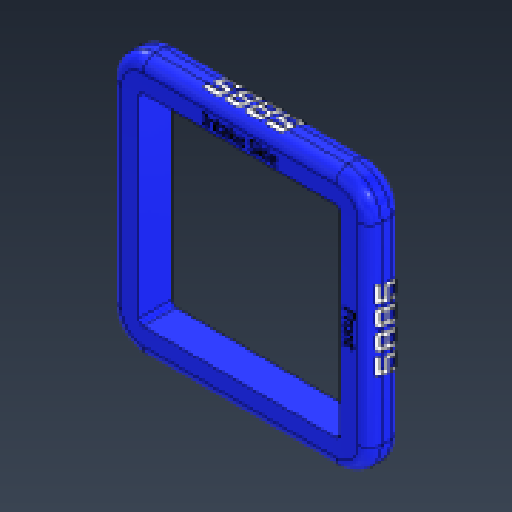
# Autodesk Inventor part: Bumpers
Saved by Autodesk Inventor 2026 (Build 300175050, 175E)
## iProperties
Created: 2026-01-21
Part Number: Bumpers
Material: Spruce
Document SubType Name: Modeling
Designer: Jthib
Mass: 13460.1 g
Surface Area: 12229.9 cm^2
Volume: 33650.4 cm^3
Density: 0.4 g/cm^3
Appearance: Blue - Wall Paint - Glossy
Author: Jthib
Autodesk Inventor part; units mm, degrees
ref_plane "YZ Plane" through (0, 0, 0) normal (1, 0, 0) x (0, 1, 0)
ref_plane "XZ Plane" through (0, 0, 0) normal (0, 1, 0) x (-1, 0, 0)
ref_plane "XY Plane" through (0, 0, 0) normal (0, 0, 1) x (1, 0, 0)
sketch "Sketch1" plane through (0, 0, 0) normal (0, 0, 1) x (1, 0, 0)
  line L0 (-349.25, 0) -> (-349.25, 336.55)
  line L1 (-336.55, 349.25) -> (336.55, 349.25)
  line L2 (349.25, 336.55) -> (349.25, -336.55)
  line L3 (336.55, -349.25) -> (-336.55, -349.25)
  line L4 (-349.25, -336.55) -> (-349.25, 0)
  arc A0 (-336.55, 349.25) -> (-349.25, 336.55) centre (-336.55, 336.55) ccw
  arc A1 (349.25, 336.55) -> (336.55, 349.25) centre (336.55, 336.55) ccw
  arc A2 (336.55, -349.25) -> (349.25, -336.55) centre (336.55, -336.55) ccw
  arc A3 (-349.25, -336.55) -> (-336.55, -349.25) centre (-336.55, -336.55) ccw
  point P0 (0, 0)
  point P1 (-349.25, 349.25)
  point P2 (349.25, 349.25)
  point P3 (349.25, -349.25)
  point P4 (-349.25, -349.25)
  dimension "d0" = 698.5
  dimension "d1" = 698.5
  dimension "d2" = 349.25
  dimension "d3" = 349.25
  dimension "d9" = 12.7
  constraints: 10 end point, 9 point on line, 8 point on circle, 8 tangent, 4 centre point, 4 perpendicular, 3 equal radius, 1 collinear, 1 vertical
  measures "d0" distance of point (349.25, 349.25) point (349.25, -349.25)
  measures "d1" distance of point (-349.25, 349.25) point (349.25, 349.25)
  measures "d2" distance from line of point (0, 0) L1
  measures "d3" distance from line of L2 point (0, 0)
  measures "d9" radius of A0
sketch "Sketch2" plane through (0, 0, 0) normal (0, 1, 0) x (-1, 0, 0)
  line L0 (412.75, 61.9125) -> (352.425, 61.9125)
  line L1 (352.425, 61.9125) -> (352.425, -52.3875)
  line L2 (352.425, -52.3875) -> (412.75, -52.3875)
  line L3 (454.025, -11.1125) -> (454.025, 20.6375)
  arc A0 (454.025, 20.6375) -> (412.75, 61.9125) centre (412.75, 20.6375) ccw
  arc A1 (412.75, -52.3875) -> (454.025, -11.1125) centre (412.75, -11.1125) ccw
  line L4 (0, -145.5372) -> (0, 106.4605) construction
  line L5 (352.425, 61.9125) -> (0, 61.9125) construction
  line L6 (352.425, -52.3875) -> (0, -52.3875) construction
  line L7 (-599.1936, -109.5375) -> (599.1891, -109.5375) construction
  point P0 (0, 0)
  point P1 (454.025, 61.9125)
  point P2 (349.25, 0)
  point P3 (349.25, 0)
  point P4 (352.425, 4.7625)
  dimension "d4" = 114.3
  dimension "d5" = 101.6
  dimension "d6" = 41.275
  dimension "d20" = 352.425
  dimension "d21" = 57.15
  constraints: 14 end point, 4 point on circle, 4 point on line, 4 tangent, 3 perpendicular, 2 centre point, 2 horizontal, 2 parallel, 1 equal radius, 1 midpoint, 2 other
  measures "d4" distance of L0.end L1.end
  measures "d5" distance of point (454.025, 61.913) L0.end
  measures "d6" radius of A0
  measures "d20" distance from line of point (0, 0) L1
  measures "d21" distance between parallel lines of L7 L2
sweep "Sweep1" add profiles "Sketch2" path "Sketch1" path curves L0 A0 L1 A1 L2 A2 L3 A3 L4
sketch "Sketch3" plane through (454.025, -336.55, 20.6375) normal (1, 0, 0) x (0, 0, -1)
  line L0 (-23.8125, 82.55) -> (-23.8125, 590.55) construction
  line L1 (-23.8125, 590.55) -> (65.0875, 590.55) construction
  line L2 (65.0875, 590.55) -> (65.0875, 82.55) construction
  line L3 (65.0875, 82.55) -> (-23.8125, 82.55) construction
  line L4 (-23.8125, 82.55) -> (65.0875, 590.55) construction
  spline S0 degree 2 poles (58.7375, 210.0554) (58.7375, 204.3206) (54.7166, 199.3768) (50.432, 199.3768) knots 0 0 0 1 2 2 2
  spline S1 degree 2 poles (50.432, 199.3768) (48.5863, 199.3768) (45.8178, 199.9701) knots 0 0 0 1 1 1
  line L5 (45.8178, 199.9701) -> (33.9527, 202.409)
  line L6 (33.9527, 202.409) -> (33.9527, 218.1632)
  line L7 (33.9527, 218.1632) -> (40.874, 216.713)
  spline S2 degree 2 poles (40.874, 216.713) (41.4013, 216.5811) (42.3242, 216.4493) (42.7856, 216.4493) knots 0 0 0 1 2 2 2
  spline S3 degree 2 poles (42.7856, 216.4493) (43.9062, 216.4493) (44.6972, 217.7017) (44.6972, 219.4156) knots 0 0 0 1 2 2 2
  line L8 (44.6972, 219.4156) -> (44.6972, 240.7727)
  spline S4 degree 2 poles (44.6972, 240.7727) (44.6972, 243.3434) (43.1152, 245.0573) (40.874, 245.6505) knots 0 0 0 1 2 2 2
  line L9 (40.874, 245.6505) -> (28.152, 248.3531)
  spline S5 degree 2 poles (28.152, 248.3531) (27.5588, 248.419) (26.7678, 248.5509) (26.4382, 248.5509) knots 0 0 0 1 2 2 2
  spline S6 degree 2 poles (26.4382, 248.5509) (24.3948, 248.5509) (24.3948, 245.6505) knots 0 0 0 1 1 1
  line L10 (24.3948, 245.6505) -> (24.3948, 204.4524)
  line L11 (24.3948, 204.4524) -> (-17.4625, 213.3512)
  line L12 (-17.4625, 213.3512) -> (-17.4625, 271.9514)
  line L13 (-17.4625, 271.9514) -> (-2.8949, 268.9192)
  line L14 (-2.8949, 268.9192) -> (-2.8949, 226.4028)
  line L15 (-2.8949, 226.4028) -> (11.8046, 223.2388)
  line L16 (11.8046, 223.2388) -> (11.8046, 257.186)
  spline S7 degree 2 poles (11.8046, 257.186) (11.8046, 261.8002) (15.7596, 266.0189) (19.3851, 266.0189) knots 0 0 0 1 2 2 2
  spline S8 degree 2 poles (19.3851, 266.0189) (20.9012, 266.0189) (22.615, 265.6234) knots 0 0 0 1 1 1
  line L17 (22.615, 265.6234) -> (45.4882, 260.8114)
  spline S9 degree 2 poles (45.4882, 260.8114) (52.2117, 259.3612) (58.7375, 252.374) (58.7375, 245.0573) knots 0 0 0 1 2 2 2
  line L18 (58.7375, 245.0573) -> (58.7375, 210.0554)
  spline S10 degree 2 poles (58.7375, 282.7618) (58.7375, 277.027) (54.7166, 271.9514) (50.432, 271.9514) knots 0 0 0 1 2 2 2
  spline S11 degree 2 poles (50.432, 271.9514) (48.5863, 271.9514) (45.8178, 272.5446) knots 0 0 0 1 1 1
  line L19 (45.8178, 272.5446) -> (27.6906, 276.3678)
  spline S12 degree 2 poles (27.6906, 276.3678) (23.406, 277.2907) (19.7147, 283.2232) (19.3851, 287.1782) knots 0 0 0 1 2 2 2
  spline S13 degree 2 poles (19.3851, 287.1782) (18.9896, 283.8824) (15.9574, 280.3228) (12.7275, 280.3228) knots 0 0 0 1 2 2 2
  spline S14 degree 2 poles (12.7275, 280.3228) (11.475, 280.3228) (9.7612, 280.6524) knots 0 0 0 1 1 1
  line L20 (9.7612, 280.6524) -> (-4.4769, 283.6846)
  spline S15 degree 2 poles (-4.4769, 283.6846) (-11.0026, 285.0689) (-17.4625, 292.5834) (-17.4625, 299.7683) knots 0 0 0 1 2 2 2
  line L21 (-17.4625, 299.7683) -> (-17.4625, 332.9905)
  spline S16 degree 2 poles (-17.4625, 332.9905) (-17.4625, 338.923) (-13.1779, 344.1304) (-8.8933, 344.1304) knots 0 0 0 1 2 2 2
  spline S17 degree 2 poles (-8.8933, 344.1304) (-6.6521, 344.1304) (-4.4769, 343.669) knots 0 0 0 1 1 1
  line L22 (-4.4769, 343.669) -> (9.7612, 340.6369)
  spline S18 degree 2 poles (9.7612, 340.6369) (14.5072, 339.5822) (18.9237, 334.1111) (19.3851, 330.0242) knots 0 0 0 1 2 2 2
  spline S19 degree 2 poles (19.3851, 330.0242) (19.7147, 333.3201) (22.4173, 337.4728) (25.4494, 337.4728) knots 0 0 0 1 2 2 2
  spline S20 degree 2 poles (25.4494, 337.4728) (25.9768, 337.4728) (27.0974, 337.341) (27.6906, 337.2751) knots 0 0 0 1 2 2 2
  line L23 (27.6906, 337.2751) -> (45.8178, 333.4519)
  spline S21 degree 2 poles (45.8178, 333.4519) (52.3436, 332.0676) (58.7375, 325.0804) (58.7375, 317.7637) knots 0 0 0 1 2 2 2
  line L24 (58.7375, 317.7637) -> (58.7375, 282.7618)
  spline S22 degree 2 poles (28.6135, 321.3891) (28.152, 321.5209) (27.361, 321.5209) knots 0 0 0 1 1 1
  spline S23 degree 2 poles (27.361, 321.5209) (26.1086, 321.5209) (25.1858, 320.0048) (25.1858, 318.0933) knots 0 0 0 1 2 2 2
  line L25 (25.1858, 318.0933) -> (25.1858, 296.6043)
  spline S24 degree 2 poles (25.1858, 296.6043) (25.1858, 294.3631) (26.6359, 292.122) (28.6135, 291.7924) knots 0 0 0 1 2 2 2
  line L26 (28.6135, 291.7924) -> (40.6103, 289.2875)
  spline S25 degree 2 poles (40.6103, 289.2875) (41.2036, 289.2216) (41.9946, 289.0898) (42.3242, 289.0898) knots 0 0 0 1 2 2 2
  spline S26 degree 2 poles (42.3242, 289.0898) (44.6972, 289.0898) (44.6972, 292.4516) knots 0 0 0 1 1 1
  line L27 (44.6972, 292.4516) -> (44.6972, 313.9405)
  spline S27 degree 2 poles (44.6972, 313.9405) (44.6972, 316.1817) (42.8515, 318.4228) (40.6103, 318.8843) knots 0 0 0 1 2 2 2
  line L28 (40.6103, 318.8843) -> (28.6135, 321.3891)
  spline S28 degree 2 poles (0.1373, 327.2557) (-0.4559, 327.3216) (-1.1151, 327.4535) (-1.4447, 327.4535) knots 0 0 0 1 2 2 2
  spline S29 degree 2 poles (-1.4447, 327.4535) (-3.6859, 327.4535) (-3.6859, 324.0917) knots 0 0 0 1 1 1
  line L29 (-3.6859, 324.0917) -> (-3.6859, 302.8005)
  spline S30 degree 2 poles (-3.6859, 302.8005) (-3.6859, 300.5593) (-2.1038, 298.5159) (0.1373, 298.1204) knots 0 0 0 1 2 2 2
  line L30 (0.1373, 298.1204) -> (10.9477, 295.8133)
  spline S31 degree 2 poles (10.9477, 295.8133) (11.3432, 295.7474) (12.0683, 295.6156) (12.3979, 295.6156) knots 0 0 0 1 2 2 2
  spline S32 degree 2 poles (12.3979, 295.6156) (14.3754, 295.6156) (14.3754, 298.8455) knots 0 0 0 1 1 1
  line L31 (14.3754, 298.8455) -> (14.3754, 320.4003)
  spline S33 degree 2 poles (14.3754, 320.4003) (14.3754, 322.6415) (12.8593, 324.5531) (10.9477, 324.9486) knots 0 0 0 1 2 2 2
  line L32 (10.9477, 324.9486) -> (0.1373, 327.2557)
  spline S34 degree 2 poles (58.7375, 355.2045) (58.7375, 349.4697) (54.7166, 344.3941) (50.432, 344.3941) knots 0 0 0 1 2 2 2
  spline S35 degree 2 poles (50.432, 344.3941) (48.5863, 344.3941) (45.8178, 344.9874) knots 0 0 0 1 1 1
  line L33 (45.8178, 344.9874) -> (27.6906, 348.8106)
  spline S36 degree 2 poles (27.6906, 348.8106) (23.406, 349.7334) (19.7147, 355.6659) (19.3851, 359.6209) knots 0 0 0 1 2 2 2
  spline S37 degree 2 poles (19.3851, 359.6209) (18.9896, 356.3251) (15.9574, 352.7656) (12.7275, 352.7656) knots 0 0 0 1 2 2 2
  spline S38 degree 2 poles (12.7275, 352.7656) (11.475, 352.7656) (9.7612, 353.0952) knots 0 0 0 1 1 1
  line L34 (9.7612, 353.0952) -> (-4.4769, 356.1273)
  spline S39 degree 2 poles (-4.4769, 356.1273) (-11.0026, 357.5116) (-17.4625, 365.0261) (-17.4625, 372.2111) knots 0 0 0 1 2 2 2
  line L35 (-17.4625, 372.2111) -> (-17.4625, 405.4332)
  spline S40 degree 2 poles (-17.4625, 405.4332) (-17.4625, 411.3657) (-13.1779, 416.5732) (-8.8933, 416.5732) knots 0 0 0 1 2 2 2
  spline S41 degree 2 poles (-8.8933, 416.5732) (-6.6521, 416.5732) (-4.4769, 416.1118) knots 0 0 0 1 1 1
  line L36 (-4.4769, 416.1118) -> (9.7612, 413.0796)
  spline S42 degree 2 poles (9.7612, 413.0796) (14.5072, 412.0249) (18.9237, 406.5538) (19.3851, 402.467) knots 0 0 0 1 2 2 2
  spline S43 degree 2 poles (19.3851, 402.467) (19.7147, 405.7628) (22.4173, 409.9156) (25.4494, 409.9156) knots 0 0 0 1 2 2 2
  spline S44 degree 2 poles (25.4494, 409.9156) (25.9768, 409.9156) (27.0974, 409.7837) (27.6906, 409.7178) knots 0 0 0 1 2 2 2
  line L37 (27.6906, 409.7178) -> (45.8178, 405.8946)
  spline S45 degree 2 poles (45.8178, 405.8946) (52.3436, 404.5104) (58.7375, 397.5232) (58.7375, 390.2064) knots 0 0 0 1 2 2 2
  line L38 (58.7375, 390.2064) -> (58.7375, 355.2045)
  spline S46 degree 2 poles (28.6135, 393.8318) (28.152, 393.9637) (27.361, 393.9637) knots 0 0 0 1 1 1
  spline S47 degree 2 poles (27.361, 393.9637) (26.1086, 393.9637) (25.1858, 392.4476) (25.1858, 390.536) knots 0 0 0 1 2 2 2
  line L39 (25.1858, 390.536) -> (25.1858, 369.0471)
  spline S48 degree 2 poles (25.1858, 369.0471) (25.1858, 366.8059) (26.6359, 364.5647) (28.6135, 364.2351) knots 0 0 0 1 2 2 2
  line L40 (28.6135, 364.2351) -> (40.6103, 361.7303)
  spline S49 degree 2 poles (40.6103, 361.7303) (41.2036, 361.6644) (41.9946, 361.5325) (42.3242, 361.5325) knots 0 0 0 1 2 2 2
  spline S50 degree 2 poles (42.3242, 361.5325) (44.6972, 361.5325) (44.6972, 364.8943) knots 0 0 0 1 1 1
  line L41 (44.6972, 364.8943) -> (44.6972, 386.3832)
  spline S51 degree 2 poles (44.6972, 386.3832) (44.6972, 388.6244) (42.8515, 390.8656) (40.6103, 391.327) knots 0 0 0 1 2 2 2
  line L42 (40.6103, 391.327) -> (28.6135, 393.8318)
  spline S52 degree 2 poles (0.1373, 399.6984) (-0.4559, 399.7644) (-1.1151, 399.8962) (-1.4447, 399.8962) knots 0 0 0 1 2 2 2
  spline S53 degree 2 poles (-1.4447, 399.8962) (-3.6859, 399.8962) (-3.6859, 396.5344) knots 0 0 0 1 1 1
  line L43 (-3.6859, 396.5344) -> (-3.6859, 375.2433)
  spline S54 degree 2 poles (-3.6859, 375.2433) (-3.6859, 373.0021) (-2.1038, 370.9586) (0.1373, 370.5631) knots 0 0 0 1 2 2 2
  line L44 (0.1373, 370.5631) -> (10.9477, 368.2561)
  spline S55 degree 2 poles (10.9477, 368.2561) (11.3432, 368.1901) (12.0683, 368.0583) (12.3979, 368.0583) knots 0 0 0 1 2 2 2
  spline S56 degree 2 poles (12.3979, 368.0583) (14.3754, 368.0583) (14.3754, 371.2882) knots 0 0 0 1 1 1
  line L45 (14.3754, 371.2882) -> (14.3754, 392.8431)
  spline S57 degree 2 poles (14.3754, 392.8431) (14.3754, 395.0843) (12.8593, 396.9958) (10.9477, 397.3913) knots 0 0 0 1 2 2 2
  line L46 (10.9477, 397.3913) -> (0.1373, 399.6984)
  spline S58 degree 2 poles (58.7375, 428.1086) (58.7375, 422.3739) (54.7166, 417.4301) (50.432, 417.4301) knots 0 0 0 1 2 2 2
  spline S59 degree 2 poles (50.432, 417.4301) (48.5863, 417.4301) (45.8178, 418.0234) knots 0 0 0 1 1 1
  line L47 (45.8178, 418.0234) -> (33.9527, 420.4623)
  line L48 (33.9527, 420.4623) -> (33.9527, 436.2164)
  line L49 (33.9527, 436.2164) -> (40.874, 434.7663)
  spline S60 degree 2 poles (40.874, 434.7663) (41.4013, 434.6344) (42.3242, 434.5026) (42.7856, 434.5026) knots 0 0 0 1 2 2 2
  spline S61 degree 2 poles (42.7856, 434.5026) (43.9062, 434.5026) (44.6972, 435.755) (44.6972, 437.4689) knots 0 0 0 1 2 2 2
  line L50 (44.6972, 437.4689) -> (44.6972, 458.8259)
  spline S62 degree 2 poles (44.6972, 458.8259) (44.6972, 461.3967) (43.1152, 463.1106) (40.874, 463.7038) knots 0 0 0 1 2 2 2
  line L51 (40.874, 463.7038) -> (28.152, 466.4064)
  spline S63 degree 2 poles (28.152, 466.4064) (27.5588, 466.4723) (26.7678, 466.6041) (26.4382, 466.6041) knots 0 0 0 1 2 2 2
  spline S64 degree 2 poles (26.4382, 466.6041) (24.3948, 466.6041) (24.3948, 463.7038) knots 0 0 0 1 1 1
  line L52 (24.3948, 463.7038) -> (24.3948, 422.5057)
  line L53 (24.3948, 422.5057) -> (-17.4625, 431.4045)
  line L54 (-17.4625, 431.4045) -> (-17.4625, 490.0047)
  line L55 (-17.4625, 490.0047) -> (-2.8949, 486.9725)
  line L56 (-2.8949, 486.9725) -> (-2.8949, 444.4561)
  line L57 (-2.8949, 444.4561) -> (11.8046, 441.292)
  line L58 (11.8046, 441.292) -> (11.8046, 475.2393)
  spline S65 degree 2 poles (11.8046, 475.2393) (11.8046, 479.8535) (15.7596, 484.0721) (19.3851, 484.0721) knots 0 0 0 1 2 2 2
  spline S66 degree 2 poles (19.3851, 484.0721) (20.9012, 484.0721) (22.615, 483.6766) knots 0 0 0 1 1 1
  line L59 (22.615, 483.6766) -> (45.4882, 478.8647)
  spline S67 degree 2 poles (45.4882, 478.8647) (52.2117, 477.4145) (58.7375, 470.4273) (58.7375, 463.1106) knots 0 0 0 1 2 2 2
  line L60 (58.7375, 463.1106) -> (58.7375, 428.1086)
  point P0 (20.6375, 336.55)
  point P1 (20.6375, 336.55)
  dimension "d0" = 698.5
  dimension "d1" = 698.5
  dimension "d2" = 349.25
  dimension "d3" = 349.25
  dimension "d9" = 12.7
  dimension "d10" = 508
  dimension "d11" = 88.9
  constraints: 2 end point, 1 coincident, 1 horizontal, 1 midpoint, 2 other
  measures "d10" distance of L0.start L0.end
  measures "d11" distance of L0.end L1.end
emboss "Emboss1" sketch "Sketch3" operation cut depth 0.254 direction (-1, 0, 0)
pattern_circular "Circular Pattern1" count 4 over 360 about axis through (0, 0, -10) along (0, 0, 1) of "Emboss1"
sketch "Sketch4" plane through (-336.55, -412.75, 61.9125) normal (0, 0, 1) x (1, 0, 0)
  line L0 (688.975, 539.75) -> (688.975, 285.75) construction
  line L1 (688.975, 285.75) -> (749.3, 285.75) construction
  line L2 (749.3, 285.75) -> (749.3, 539.75) construction
  line L3 (749.3, 539.75) -> (688.975, 539.75) construction
  line L4 (688.975, 749.3) -> (688.975, 76.2) projected
  line L5 (749.3, 749.3) -> (749.3, 76.2) projected
  line L6 (734.0811, 446.8053) -> (734.0811, 464.5277)
  line L7 (734.0811, 464.5277) -> (723.3365, 464.5277)
  line L8 (723.3365, 464.5277) -> (723.3365, 447.5464)
  line L9 (723.3365, 447.5464) -> (718.8287, 447.5464)
  line L10 (718.8287, 447.5464) -> (718.8287, 464.5277)
  line L11 (718.8287, 464.5277) -> (700.4889, 464.5277)
  line L12 (700.4889, 464.5277) -> (700.4889, 469.5912)
  line L13 (700.4889, 469.5912) -> (738.5889, 469.5912)
  line L14 (738.5889, 469.5912) -> (738.5889, 446.8053)
  line L15 (738.5889, 446.8053) -> (734.0811, 446.8053)
  line L16 (723.9232, 427.4775) -> (723.9232, 427.7245)
  spline S0 degree 2 poles (723.9232, 427.7245) (724.0775, 428.2802) (724.1393, 429.4844) (724.1393, 430.318) knots 0 0 0 1 2 2 2
  spline S1 degree 2 poles (724.1393, 430.318) (724.1393, 432.2631) (722.4411, 436.0917) (720.7739, 437.8207) knots 0 0 0 1 2 2 2
  line L17 (720.7739, 437.8207) -> (700.4889, 437.8207)
  line L18 (700.4889, 437.8207) -> (700.4889, 442.6372)
  line L19 (700.4889, 442.6372) -> (729.0793, 442.6372)
  line L20 (729.0793, 442.6372) -> (729.0793, 437.8207)
  line L21 (729.0793, 437.8207) -> (724.8185, 437.8207)
  spline S2 degree 2 poles (724.8185, 437.8207) (727.1651, 435.1963) (729.0793, 431.2751) (729.0793, 429.4226) knots 0 0 0 1 2 2 2
  spline S3 degree 2 poles (729.0793, 429.4226) (729.0793, 428.6816) (729.0176, 427.9406) (728.9249, 427.4775) knots 0 0 0 1 2 2 2
  line L22 (728.9249, 427.4775) -> (723.9232, 427.4775)
  spline S4 degree 2 poles (714.7841, 400.2455) (707.5593, 400.2455) (699.6861, 407.1925) (699.6861, 412.997) knots 0 0 0 1 2 2 2
  spline S5 degree 2 poles (699.6861, 412.997) (699.6861, 418.9559) (707.8063, 425.7793) (714.7841, 425.7793) knots 0 0 0 1 2 2 2
  spline S6 degree 2 poles (714.7841, 425.7793) (721.9471, 425.7793) (729.8821, 418.7398) (729.8821, 412.997) knots 0 0 0 1 2 2 2
  spline S7 degree 2 poles (729.8821, 412.997) (729.8821, 407.1925) (721.978, 400.2455) (714.7841, 400.2455) knots 0 0 0 1 2 2 2
  spline S8 degree 2 poles (714.7841, 405.2164) (720.3416, 405.2164) (725.7448, 409.2611) (725.7448, 412.997) knots 0 0 0 1 2 2 2
  spline S9 degree 2 poles (725.7448, 412.997) (725.7448, 416.7329) (720.3416, 420.8084) (714.7841, 420.8084) knots 0 0 0 1 2 2 2
  spline S10 degree 2 poles (714.7841, 420.8084) (709.3809, 420.8084) (703.8234, 416.7329) (703.8234, 412.997) knots 0 0 0 1 2 2 2
  spline S11 degree 2 poles (703.8234, 412.997) (703.8234, 409.292) (709.2883, 405.2164) (714.7841, 405.2164) knots 0 0 0 1 2 2 2
  line L23 (700.4889, 372.8592) -> (700.4889, 377.6758)
  line L24 (700.4889, 377.6758) -> (716.791, 377.6758)
  spline S12 degree 2 poles (716.791, 377.6758) (718.767, 377.6758) (722.1633, 378.0463) (723.1822, 378.602) knots 0 0 0 1 2 2 2
  spline S13 degree 2 poles (723.1822, 378.602) (724.2628, 379.1887) (725.3125, 381.2882) (725.3125, 383.0789) knots 0 0 0 1 2 2 2
  spline S14 degree 2 poles (725.3125, 383.0789) (725.3125, 384.8697) (723.3983, 388.6673) (721.8545, 390.489) knots 0 0 0 1 2 2 2
  line L25 (721.8545, 390.489) -> (700.4889, 390.489)
  line L26 (700.4889, 390.489) -> (700.4889, 395.3055)
  line L27 (700.4889, 395.3055) -> (729.0793, 395.3055)
  line L28 (729.0793, 395.3055) -> (729.0793, 390.489)
  line L29 (729.0793, 390.489) -> (725.8992, 390.489)
  spline S15 degree 2 poles (725.8992, 390.489) (727.8443, 388.3277) (729.8821, 384.1596) (729.8821, 381.813) knots 0 0 0 1 2 2 2
  spline S16 degree 2 poles (729.8821, 381.813) (729.8821, 377.614) (724.3245, 372.8592) (719.0449, 372.8592) knots 0 0 0 1 2 2 2
  line L30 (719.0449, 372.8592) -> (700.4889, 372.8592)
  spline S17 degree 2 poles (699.9331, 357.4525) (699.9331, 361.3737) (704.41, 365.7888) (709.2574, 365.7888) knots 0 0 0 1 2 2 2
  line L31 (709.2574, 365.7888) -> (725.0964, 365.7888)
  line L32 (725.0964, 365.7888) -> (725.0964, 369.0307)
  line L33 (725.0964, 369.0307) -> (729.0793, 369.0307)
  line L34 (729.0793, 369.0307) -> (729.0793, 365.7888)
  line L35 (729.0793, 365.7888) -> (737.2921, 365.7888)
  line L36 (737.2921, 365.7888) -> (737.2921, 360.9723)
  line L37 (737.2921, 360.9723) -> (729.0793, 360.9723)
  line L38 (729.0793, 360.9723) -> (729.0793, 352.1111)
  line L39 (729.0793, 352.1111) -> (725.0964, 352.1111)
  line L40 (725.0964, 352.1111) -> (725.0964, 360.9723)
  line L41 (725.0964, 360.9723) -> (711.4804, 360.9723)
  spline S18 degree 2 poles (711.4804, 360.9723) (709.3192, 360.9723) (706.9418, 360.8179) (705.9229, 360.293) knots 0 0 0 1 2 2 2
  spline S19 degree 2 poles (705.9229, 360.293) (705.0275, 359.8608) (704.1322, 357.9156) (704.1322, 356.2484) knots 0 0 0 1 2 2 2
  spline S20 degree 2 poles (704.1322, 356.2484) (704.1322, 355.0751) (704.8423, 352.883) (705.0584, 352.389) knots 0 0 0 1 2 2 2
  line L42 (705.0584, 352.389) -> (705.0584, 352.1111)
  line L43 (705.0584, 352.1111) -> (700.7359, 352.1111)
  spline S21 degree 2 poles (700.7359, 352.1111) (700.3654, 353.4696) (699.9331, 356.2484) (699.9331, 357.4525) knots 0 0 0 1 2 2 2
  point P0 (336.55, 412.75)
  point P1 (749.3, 412.75)
  dimension "d0" = 698.5
  dimension "d1" = 698.5
  dimension "d2" = 349.25
  dimension "d3" = 349.25
  dimension "d9" = 12.7
  dimension "d17" = 254
  constraints: 2 midpoint, 1 collinear, 2 other
  measures "d17" distance between parallel lines of L1 L3
emboss "Emboss2" sketch "Sketch4" operation cut depth 0.254 direction (0, 0, -1)
sketch "Sketch5" plane through (-336.55, -412.75, 61.9125) normal (0, 0, 1) x (1, 0, 0)
  line L0 (0, 825.5) -> (673.1, 825.5) construction
  line L1 (673.1, 825.5) -> (673.1, 765.175) construction
  line L2 (673.1, 765.175) -> (0, 765.175) construction
  line L3 (0, 765.175) -> (0, 825.5) construction
  line L4 (0, 825.5) -> (673.1, 825.5) construction
  line L5 (0, 765.175) -> (673.1, 765.175) construction
  line L6 (336.55, -222.8958) -> (336.55, 1048.3958) construction
  line L7 (222.9293, 775.8398) -> (208.1709, 775.8398)
  line L8 (208.1709, 775.8398) -> (208.1709, 779.7301)
  line L9 (208.1709, 779.7301) -> (213.0183, 779.7301)
  line L10 (213.0183, 779.7301) -> (213.0183, 810.0495)
  line L11 (213.0183, 810.0495) -> (208.1709, 810.0495)
  line L12 (208.1709, 810.0495) -> (208.1709, 813.9398)
  line L13 (208.1709, 813.9398) -> (222.9293, 813.9398)
  line L14 (222.9293, 813.9398) -> (222.9293, 810.0495)
  line L15 (222.9293, 810.0495) -> (218.0819, 810.0495)
  line L16 (218.0819, 810.0495) -> (218.0819, 779.7301)
  line L17 (218.0819, 779.7301) -> (222.9293, 779.7301)
  line L18 (222.9293, 779.7301) -> (222.9293, 775.8398)
  line L19 (251.2727, 775.8398) -> (246.4562, 775.8398)
  line L20 (246.4562, 775.8398) -> (246.4562, 792.1419)
  spline S0 degree 2 poles (246.4562, 792.1419) (246.4562, 794.1179) (246.0857, 797.5142) (245.5299, 798.5331) knots 0 0 0 1 2 2 2
  spline S1 degree 2 poles (245.5299, 798.5331) (244.9433, 799.6137) (242.8438, 800.6635) (241.053, 800.6635) knots 0 0 0 1 2 2 2
  spline S2 degree 2 poles (241.053, 800.6635) (239.2622, 800.6635) (235.4646, 798.7492) (233.643, 797.2055) knots 0 0 0 1 2 2 2
  line L21 (233.643, 797.2055) -> (233.643, 775.8398)
  line L22 (233.643, 775.8398) -> (228.8264, 775.8398)
  line L23 (228.8264, 775.8398) -> (228.8264, 804.4302)
  line L24 (228.8264, 804.4302) -> (233.643, 804.4302)
  line L25 (233.643, 804.4302) -> (233.643, 801.2501)
  spline S3 degree 2 poles (233.643, 801.2501) (235.8042, 803.1952) (239.9724, 805.233) (242.3189, 805.233) knots 0 0 0 1 2 2 2
  spline S4 degree 2 poles (242.3189, 805.233) (246.5179, 805.233) (251.2727, 799.6755) (251.2727, 794.3958) knots 0 0 0 1 2 2 2
  line L26 (251.2727, 794.3958) -> (251.2727, 775.8398)
  spline S5 degree 2 poles (266.6794, 775.2841) (262.7583, 775.2841) (258.3431, 779.761) (258.3431, 784.6084) knots 0 0 0 1 2 2 2
  line L27 (258.3431, 784.6084) -> (258.3431, 800.4473)
  line L28 (258.3431, 800.4473) -> (255.1012, 800.4473)
  line L29 (255.1012, 800.4473) -> (255.1012, 804.4302)
  line L30 (255.1012, 804.4302) -> (258.3431, 804.4302)
  line L31 (258.3431, 804.4302) -> (258.3431, 812.6431)
  line L32 (258.3431, 812.6431) -> (263.1597, 812.6431)
  line L33 (263.1597, 812.6431) -> (263.1597, 804.4302)
  line L34 (263.1597, 804.4302) -> (272.0208, 804.4302)
  line L35 (272.0208, 804.4302) -> (272.0208, 800.4473)
  line L36 (272.0208, 800.4473) -> (263.1597, 800.4473)
  line L37 (263.1597, 800.4473) -> (263.1597, 786.8314)
  spline S6 degree 2 poles (263.1597, 786.8314) (263.1597, 784.6701) (263.314, 782.2927) (263.8389, 781.2738) knots 0 0 0 1 2 2 2
  spline S7 degree 2 poles (263.8389, 781.2738) (264.2712, 780.3785) (266.2163, 779.4831) (267.8836, 779.4831) knots 0 0 0 1 2 2 2
  spline S8 degree 2 poles (267.8836, 779.4831) (269.0568, 779.4831) (271.249, 780.1932) (271.743, 780.4093) knots 0 0 0 1 2 2 2
  line L38 (271.743, 780.4093) -> (272.0208, 780.4093)
  line L39 (272.0208, 780.4093) -> (272.0208, 776.0868)
  spline S9 degree 2 poles (272.0208, 776.0868) (270.6623, 775.7163) (267.8836, 775.2841) (266.6794, 775.2841) knots 0 0 0 1 2 2 2
  spline S10 degree 2 poles (291.5031, 778.8656) (290.9165, 778.4333) (288.9404, 776.8896) (288.0142, 776.4264) knots 0 0 0 1 2 2 2
  spline S11 degree 2 poles (288.0142, 776.4264) (286.7483, 775.7472) (284.3709, 775.0371) (282.2097, 775.0371) knots 0 0 0 1 2 2 2
  spline S12 degree 2 poles (282.2097, 775.0371) (280.4498, 775.0371) (277.2696, 776.3647) (276.0655, 777.5688) knots 0 0 0 1 2 2 2
  spline S13 degree 2 poles (276.0655, 777.5688) (274.9231, 778.7421) (273.5337, 782.2001) (273.5337, 784.1144) knots 0 0 0 1 2 2 2
  spline S14 degree 2 poles (273.5337, 784.1144) (273.5337, 787.0784) (276.0346, 791.2774) (278.7516, 792.4815) knots 0 0 0 1 2 2 2
  spline S15 degree 2 poles (278.7516, 792.4815) (281.1599, 793.5931) (287.7054, 794.4267) (291.5031, 794.6428) knots 0 0 0 1 2 2 2
  line L40 (291.5031, 794.6428) -> (291.5031, 795.5691)
  spline S16 degree 2 poles (291.5031, 795.5691) (291.5031, 797.2363) (290.4842, 799.305) (289.5579, 799.8916) knots 0 0 0 1 2 2 2
  spline S17 degree 2 poles (289.5579, 799.8916) (288.6317, 800.4782) (285.9764, 800.8487) (284.5562, 800.8487) knots 0 0 0 1 2 2 2
  spline S18 degree 2 poles (284.5562, 800.8487) (282.8889, 800.8487) (278.3811, 799.8607) (276.1272, 798.9036) knots 0 0 0 1 2 2 2
  line L41 (276.1272, 798.9036) -> (275.8494, 798.9036)
  line L42 (275.8494, 798.9036) -> (275.8494, 803.8127)
  spline S19 degree 2 poles (275.8494, 803.8127) (277.177, 804.1832) (282.1479, 805.1095) (284.587, 805.1095) knots 0 0 0 1 2 2 2
  spline S20 degree 2 poles (284.587, 805.1095) (287.5511, 805.1095) (291.5957, 804.1832) (293.2012, 802.9791) knots 0 0 0 1 2 2 2
  spline S21 degree 2 poles (293.2012, 802.9791) (294.7759, 801.8059) (296.3196, 798.07) (296.3196, 795.3838) knots 0 0 0 1 2 2 2
  line L43 (296.3196, 795.3838) -> (296.3196, 775.8398)
  line L44 (296.3196, 775.8398) -> (291.5031, 775.8398)
  line L45 (291.5031, 775.8398) -> (291.5031, 778.8656)
  line L46 (291.5031, 782.8794) -> (291.5031, 790.8143)
  spline S22 degree 2 poles (291.5031, 790.8143) (289.7741, 790.6599) (284.5562, 790.135) (282.9198, 789.641) knots 0 0 0 1 2 2 2
  spline S23 degree 2 poles (282.9198, 789.641) (281.0055, 789.0544) (278.5046, 786.6153) (278.5046, 784.454) knots 0 0 0 1 2 2 2
  spline S24 degree 2 poles (278.5046, 784.454) (278.5046, 781.984) (281.2834, 779.4831) (283.9387, 779.4831) knots 0 0 0 1 2 2 2
  spline S25 degree 2 poles (283.9387, 779.4831) (286.1926, 779.4831) (289.8976, 781.4282) (291.5031, 782.8794) knots 0 0 0 1 2 2 2
  line L47 (326.7626, 775.8398) -> (320.4332, 775.8398)
  line L48 (320.4332, 775.8398) -> (309.8121, 789.641)
  line L49 (309.8121, 789.641) -> (307.8978, 787.7885)
  line L50 (307.8978, 787.7885) -> (307.8978, 775.8398)
  line L51 (307.8978, 775.8398) -> (303.0813, 775.8398)
  line L52 (303.0813, 775.8398) -> (303.0813, 815.6379)
  line L53 (303.0813, 815.6379) -> (307.8978, 815.6379)
  line L54 (307.8978, 815.6379) -> (307.8978, 792.358)
  line L55 (307.8978, 792.358) -> (319.1981, 804.4302)
  line L56 (319.1981, 804.4302) -> (325.1879, 804.4302)
  line L57 (325.1879, 804.4302) -> (313.4554, 792.4815)
  line L58 (313.4554, 792.4815) -> (326.7626, 775.8398)
  spline S26 degree 2 poles (341.5827, 775.1914) (334.7284, 775.1914) (327.1948, 782.8794) (327.1948, 789.9807) knots 0 0 0 1 2 2 2
  spline S27 degree 2 poles (327.1948, 789.9807) (327.1948, 796.9584) (334.5122, 805.233) (340.4094, 805.233) knots 0 0 0 1 2 2 2
  spline S28 degree 2 poles (340.4094, 805.233) (343.0647, 805.233) (347.1711, 803.6892) (348.684, 802.0529) knots 0 0 0 1 2 2 2
  spline S29 degree 2 poles (348.684, 802.0529) (350.2277, 800.4165) (351.8641, 795.6926) (351.8641, 792.2654) knots 0 0 0 1 2 2 2
  line L59 (351.8641, 792.2654) -> (351.8641, 789.641)
  line L60 (351.8641, 789.641) -> (332.0731, 789.641)
  spline S30 degree 2 poles (332.0731, 789.641) (332.0731, 784.6701) (337.0749, 779.3905) (341.5209, 779.3905) knots 0 0 0 1 2 2 2
  spline S31 degree 2 poles (341.5209, 779.3905) (343.0956, 779.3905) (346.1522, 780.1006) (347.3872, 780.6563) knots 0 0 0 1 2 2 2
  spline S32 degree 2 poles (347.3872, 780.6563) (348.684, 781.2738) (350.4747, 782.3545) (351.0614, 782.8485) knots 0 0 0 1 2 2 2
  line L61 (351.0614, 782.8485) -> (351.3392, 782.8485)
  line L62 (351.3392, 782.8485) -> (351.3392, 777.5997)
  spline S33 degree 2 poles (351.3392, 777.5997) (350.5056, 777.2601) (347.9738, 776.2721) (346.9858, 775.9942) knots 0 0 0 1 2 2 2
  spline S34 degree 2 poles (346.9858, 775.9942) (345.5964, 775.5928) (343.3117, 775.1914) (341.5827, 775.1914) knots 0 0 0 1 2 2 2
  spline S35 degree 2 poles (347.1711, 793.3152) (347.1093, 795.2603) (346.3066, 798.1008) (345.5347, 799.058) knots 0 0 0 1 2 2 2
  spline S36 degree 2 poles (345.5347, 799.058) (344.7011, 800.1386) (342.0767, 801.281) (340.1315, 801.281) knots 0 0 0 1 2 2 2
  spline S37 degree 2 poles (340.1315, 801.281) (338.2173, 801.281) (335.5311, 800.1386) (334.4196, 799.0271) knots 0 0 0 1 2 2 2
  spline S38 degree 2 poles (334.4196, 799.0271) (333.339, 797.8847) (332.2275, 795.1368) (332.0731, 793.3152) knots 0 0 0 1 2 2 2
  line L63 (332.0731, 793.3152) -> (347.1711, 793.3152)
  spline S39 degree 2 poles (384.0978, 775.1606) (379.9605, 775.1606) (374.156, 776.8896) (371.5934, 778.1246) knots 0 0 0 1 2 2 2
  line L64 (371.5934, 778.1246) -> (371.5934, 784.4849)
  line L65 (371.5934, 784.4849) -> (371.9639, 784.4849)
  spline S40 degree 2 poles (371.9639, 784.4849) (374.4648, 782.1384) (380.7942, 779.5448) (383.7273, 779.5448) knots 0 0 0 1 2 2 2
  spline S41 degree 2 poles (383.7273, 779.5448) (387.9263, 779.5448) (392.218, 783.0337) (392.218, 785.9051) knots 0 0 0 1 2 2 2
  spline S42 degree 2 poles (392.218, 785.9051) (392.218, 788.1899) (389.9641, 791.0304) (387.525, 791.7405) knots 0 0 0 1 2 2 2
  spline S43 degree 2 poles (387.525, 791.7405) (385.7651, 792.2345) (382.8319, 792.9138) (380.6398, 793.4696) knots 0 0 0 1 2 2 2
  spline S44 degree 2 poles (380.6398, 793.4696) (378.6638, 793.9944) (375.5454, 795.5691) (374.3413, 796.8349) knots 0 0 0 1 2 2 2
  spline S45 degree 2 poles (374.3413, 796.8349) (373.168, 798.1008) (371.8712, 801.4971) (371.8712, 803.7201) knots 0 0 0 1 2 2 2
  spline S46 degree 2 poles (371.8712, 803.7201) (371.8712, 808.3514) (379.096, 814.6191) (384.6844, 814.6191) knots 0 0 0 1 2 2 2
  spline S47 degree 2 poles (384.6844, 814.6191) (387.8955, 814.6191) (393.5765, 813.3532) (396.0156, 812.149) knots 0 0 0 1 2 2 2
  line L66 (396.0156, 812.149) -> (396.0156, 806.0975)
  line L67 (396.0156, 806.0975) -> (395.6451, 806.0975)
  spline S48 degree 2 poles (395.6451, 806.0975) (393.8235, 807.7648) (388.1425, 810.2348) (385.0241, 810.2348) knots 0 0 0 1 2 2 2
  spline S49 degree 2 poles (385.0241, 810.2348) (381.5043, 810.2348) (377.1509, 806.9311) (377.1509, 804.245) knots 0 0 0 1 2 2 2
  spline S50 degree 2 poles (377.1509, 804.245) (377.1509, 801.8367) (379.7135, 798.9653) (382.1218, 798.317) knots 0 0 0 1 2 2 2
  spline S51 degree 2 poles (382.1218, 798.317) (383.7273, 797.8847) (388.3895, 796.7732) (389.9332, 796.3101) knots 0 0 0 1 2 2 2
  spline S52 degree 2 poles (389.9332, 796.3101) (393.8544, 795.1059) (397.4977, 790.2585) (397.4977, 786.7079) knots 0 0 0 1 2 2 2
  spline S53 degree 2 poles (397.4977, 786.7079) (397.4977, 784.454) (395.676, 780.1315) (394.0396, 778.6186) knots 0 0 0 1 2 2 2
  spline S54 degree 2 poles (394.0396, 778.6186) (392.218, 776.9513) (387.5867, 775.1606) (384.0978, 775.1606) knots 0 0 0 1 2 2 2
  line L68 (407.1925, 775.8398) -> (402.3759, 775.8398)
  line L69 (402.3759, 775.8398) -> (402.3759, 804.4302)
  line L70 (402.3759, 804.4302) -> (407.1925, 804.4302)
  line L71 (407.1925, 804.4302) -> (407.1925, 775.8398)
  line L72 (407.5321, 809.185) -> (402.0672, 809.185)
  line L73 (402.0672, 809.185) -> (402.0672, 814.1868)
  line L74 (402.0672, 814.1868) -> (407.5321, 814.1868)
  line L75 (407.5321, 814.1868) -> (407.5321, 809.185)
  line L76 (436.246, 775.8398) -> (431.4295, 775.8398)
  line L77 (431.4295, 775.8398) -> (431.4295, 778.7421)
  spline S55 degree 2 poles (431.4295, 778.7421) (430.318, 777.8158) (428.6816, 776.5808) (427.5701, 776.0559) knots 0 0 0 1 2 2 2
  spline S56 degree 2 poles (427.5701, 776.0559) (426.5512, 775.5619) (424.3591, 775.0371) (422.9079, 775.0371) knots 0 0 0 1 2 2 2
  spline S57 degree 2 poles (422.9079, 775.0371) (420.5614, 775.0371) (416.6094, 776.9822) (415.22, 778.8656) knots 0 0 0 1 2 2 2
  spline S58 degree 2 poles (415.22, 778.8656) (413.8306, 780.749) (412.2869, 786.3065) (412.2869, 789.9189) knots 0 0 0 1 2 2 2
  spline S59 degree 2 poles (412.2869, 789.9189) (412.2869, 793.6857) (414.232, 799.1815) (415.9302, 801.2501) knots 0 0 0 1 2 2 2
  spline S60 degree 2 poles (415.9302, 801.2501) (417.5048, 803.1026) (421.9199, 805.233) (424.3591, 805.233) knots 0 0 0 1 2 2 2
  spline S61 degree 2 poles (424.3591, 805.233) (426.4895, 805.233) (429.6696, 804.2759) (431.4295, 803.2879) knots 0 0 0 1 2 2 2
  line L78 (431.4295, 803.2879) -> (431.4295, 815.6379)
  line L79 (431.4295, 815.6379) -> (436.246, 815.6379)
  line L80 (436.246, 815.6379) -> (436.246, 775.8398)
  line L81 (431.4295, 782.7867) -> (431.4295, 799.305)
  spline S62 degree 2 poles (431.4295, 799.305) (429.6387, 800.1695) (426.7982, 800.8178) (425.1618, 800.8178) knots 0 0 0 1 2 2 2
  spline S63 degree 2 poles (425.1618, 800.8178) (421.4568, 800.8178) (417.2578, 795.2603) (417.2578, 790.0115) knots 0 0 0 1 2 2 2
  spline S64 degree 2 poles (417.2578, 790.0115) (417.2578, 784.948) (420.4688, 779.6066) (424.0195, 779.6066) knots 0 0 0 1 2 2 2
  spline S65 degree 2 poles (424.0195, 779.6066) (425.9028, 779.6066) (429.7314, 781.3356) (431.4295, 782.7867) knots 0 0 0 1 2 2 2
  spline S66 degree 2 poles (455.6357, 775.1914) (448.7814, 775.1914) (441.2478, 782.8794) (441.2478, 789.9807) knots 0 0 0 1 2 2 2
  spline S67 degree 2 poles (441.2478, 789.9807) (441.2478, 796.9584) (448.5652, 805.233) (454.4624, 805.233) knots 0 0 0 1 2 2 2
  spline S68 degree 2 poles (454.4624, 805.233) (457.1177, 805.233) (461.2241, 803.6892) (462.737, 802.0529) knots 0 0 0 1 2 2 2
  spline S69 degree 2 poles (462.737, 802.0529) (464.2807, 800.4165) (465.9171, 795.6926) (465.9171, 792.2654) knots 0 0 0 1 2 2 2
  line L82 (465.9171, 792.2654) -> (465.9171, 789.641)
  line L83 (465.9171, 789.641) -> (446.1261, 789.641)
  spline S70 degree 2 poles (446.1261, 789.641) (446.1261, 784.6701) (451.1279, 779.3905) (455.5739, 779.3905) knots 0 0 0 1 2 2 2
  spline S71 degree 2 poles (455.5739, 779.3905) (457.1485, 779.3905) (460.2052, 780.1006) (461.4402, 780.6563) knots 0 0 0 1 2 2 2
  spline S72 degree 2 poles (461.4402, 780.6563) (462.737, 781.2738) (464.5277, 782.3545) (465.1143, 782.8485) knots 0 0 0 1 2 2 2
  line L84 (465.1143, 782.8485) -> (465.3922, 782.8485)
  line L85 (465.3922, 782.8485) -> (465.3922, 777.5997)
  spline S73 degree 2 poles (465.3922, 777.5997) (464.5586, 777.2601) (462.0268, 776.2721) (461.0388, 775.9942) knots 0 0 0 1 2 2 2
  spline S74 degree 2 poles (461.0388, 775.9942) (459.6494, 775.5928) (457.3647, 775.1914) (455.6357, 775.1914) knots 0 0 0 1 2 2 2
  spline S75 degree 2 poles (461.2241, 793.3152) (461.1623, 795.2603) (460.3596, 798.1008) (459.5877, 799.058) knots 0 0 0 1 2 2 2
  spline S76 degree 2 poles (459.5877, 799.058) (458.7541, 800.1386) (456.1297, 801.281) (454.1845, 801.281) knots 0 0 0 1 2 2 2
  spline S77 degree 2 poles (454.1845, 801.281) (452.2703, 801.281) (449.5841, 800.1386) (448.4726, 799.0271) knots 0 0 0 1 2 2 2
  spline S78 degree 2 poles (448.4726, 799.0271) (447.392, 797.8847) (446.2805, 795.1368) (446.1261, 793.3152) knots 0 0 0 1 2 2 2
  line L86 (446.1261, 793.3152) -> (461.2241, 793.3152)
  point P0 (336.55, 412.75)
  point P1 (336.55, 765.175)
  dimension "d0" = 698.5
  dimension "d1" = 698.5
  dimension "d2" = 349.25
  dimension "d3" = 349.25
  dimension "d9" = 12.7
  constraints: 3 collinear, 1 midpoint, 1 point on line, 2 other
emboss "Emboss3" sketch "Sketch5" operation cut depth 0.254 direction (0, 0, -1)
equation "\"d0\" = d1"
equation "\"d2\" = 0.5 * d0"
equation "\"d3\" = 0.5 * d1"
body "Solid1"
